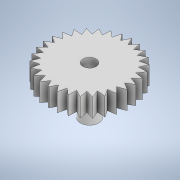
# Autodesk Inventor part: motor driven gear straight teeth for potentiometer
Saved by Autodesk Inventor 2022 (Build 260153000, 153)
## iProperties
Created: 2021-11-09
Part Number: motor driven gear straight teeth for potentiometer
Material: Generic
Document SubType Name: Modeling
Designer: a-dubs
Density: 1 g/cm^3
Appearance: Default
Author: a-dubs
Autodesk Inventor part; units mm, degrees
ref_plane "YZ Plane" through (0, 0, 0) normal (1, 0, 0) x (0, 1, 0)
ref_plane "XZ Plane" through (0, 0, 0) normal (0, 1, 0) x (-1, 0, 0)
ref_plane "XY Plane" through (0, 0, 0) normal (0, 0, 1) x (1, 0, 0)
sketch "Sketch1" plane through (0, 0, 0) normal (0, 1, 0) x (-1, 0, 0)
  line L0 (-2, 0) -> (2, 0)
  line L1 (-2, 0) -> (-2, 1)
  line L2 (-2, 1) -> (0, 0)
  line L3 (0, 0) -> (2, 1)
  line L4 (0, 0) -> (0, 19)
  line L5 (0, 19) -> (2, 19)
  line L6 (-2, 19) -> (0, 19)
  line L7 (0, 19) -> (0, 23)
  line L8 (0, 23) -> (-2, 19)
  line L9 (2, 19) -> (0, 23)
  line L10 (2, 0) -> (2, 19)
  line L11 (-2, 19) -> (-2, 0)
  point P0 (0, 41)
  dimension "d6" = 1
  dimension "d10" = 19
  dimension "d11" = 4
  constraints: 24 end point, 2 equal length, 1 vertical
  measures "d6" distance of L0.start L1.end
  measures "d10" distance of L2.end L4.end
  measures "d11" distance of L4.end L7.end
extrude "Extrusion1" add sketch "Sketch1" along normal blind 26 contours L3 L10 L0 | L4 L5 L10 L3 | L2 L11 L6 L4 | L7 L9 L5 | L6 L8 L7
pattern_circular "Circular Pattern1" count 30 over 360 about axis through (0, 0, 0) along (0, 1, 0) of "Extrusion1"
fillet "Fillet1" radius 0.5 1 edges at (0, 13, 23)
sketch "Sketch2" plane through (0, 26, 0) normal (0, 1, 0) x (1, 0, 0)
  circle A0 centre (0, 0) radius 1.5
  circle A1 centre (0, 0) radius 2.8
  line L0 (0, 0) -> (0, 1.9)
  line L1 (0, 1.9) -> (0, -1.9)
  line L2 (0, -1.9) -> (-2.0567, -1.9)
  line L3 (0, -1.9) -> (2.0567, -1.9)
  line L4 (0, 1.9) -> (2.0567, 1.9)
  line L5 (0, 1.9) -> (-2.0567, 1.9)
  circle A2 centre (0, 0) radius 3.6
  line L6 (0, 0) -> (0, 0.7)
  line L7 (0, 0) -> (0, -0.7)
  circle A3 centre (0, 0) radius 2.9
  line L8 (0, 0.7) -> (-2.8142, 0.7)
  line L9 (0, -0.7) -> (-2.8142, -0.7)
  line L10 (0, -0.7) -> (2.8142, -0.7)
  line L11 (0, 0.7) -> (2.8142, 0.7)
  circle A4 centre (0, 0) radius 5
  circle A5 centre (0, 0) radius 15
  circle A6 centre (0, 0) radius 30.1844
  line L12 (-2.0567, 1.9) -> (-2.1909, 1.9)
  line L13 (-2.1909, -1.9) -> (-2.0567, -1.9)
  line L14 (2.0567, -1.9) -> (2.1909, -1.9)
  line L15 (2.0567, 1.9) -> (2.1909, 1.9)
  line L16 (-1.0864, -1.9) -> (-1.0864, -2)
  line L17 (-1.0864, 1.9) -> (-1.0864, 2)
  line L18 (-1.0864, 2) -> (-2.1, 2)
  line L19 (-1.0864, 2) -> (2.1, 2)
  line L20 (-2.1, -2) -> (-1.0864, -2)
  line L21 (-1.0864, -2) -> (2.1, -2)
  circle A7 centre (0, 0) radius 3
  point P0 (1.9596, -2)
  point P1 (-1.9596, -2)
  point P2 (1.9596, 2)
  point P3 (-1.9596, 2)
  dimension "d30" = 5.8
  dimension "d13" = 3
  dimension "d19" = 5.6
  dimension "d20" = 1.9
  dimension "d21" = 3.8
  dimension "d27" = 7.2
  dimension "d28" = 0.7
  dimension "d29" = 0.7
  dimension "d37" = 10
  dimension "d38" = 30
  dimension "d43" = 0.1
  dimension "d44" = 0.1
  dimension "d47" = 6
  constraints: 44 end point, 11 point on line, 8 coincident, 7 centre point, 5 parallel, 4 point on circle, 3 horizontal, 3 vertical, 1 perpendicular, 14 other
  measures "d13" diameter of A0
  measures "d19" diameter of A1
  measures "d20" distance of L0.start L0.end
  measures "d21" distance of L0.end L1.end
  measures "d27" diameter of A2
  measures "d28" distance of L6.start L6.end
  measures "d29" distance of L6.start L7.end
  measures "d37" diameter of A4
  measures "d38" diameter of A5
  measures "d43" distance of L16.start L16.end
  measures "d44" distance of L17.start L17.end
  measures "d47" diameter of A7
extrude "Extrusion2" cut sketch "Sketch2" against normal blind 7.5 contours A0 L10 L1 L0 L11 | A0 L11 A1 L10 | L11 L0 A0 | A0 L0 L4 A1 L11 | L10 A1 L3 L1 A0 | A0 L1 L10 | L0 L8 A0 | A0 L8 A1 L5 L0 | L0 L1 L9 A0 L8 | L11 A3 L10 A1 | A1 L15 A3 L11 | L1 L2 A1 L9 A0 | A0 L9 L1 | L10 A3 L14 A1 | A0 L9 A1 L8 | L5 L17 L19 A1 L4 | A1 L19 A3 L15 | L3 A1 L21 L16 L2 | L14 A3 L21 A1 | L8 A3 L12 A1 | A1 L9 A3 L8 | L5 A1 L18 L17 | L19 L18 A1 | A1 L18 A3 L19 | A1 L13 A3 L9 | L16 L20 A1 L2 | L21 A3 L20 A1 | A1 L20 L21 | L12 A3 L18 A1 | A1 L20 A3 L13 | A2 | A7
pattern_circular "Circular Pattern2" [suppressed]
extrude "Extrusion4" cut sketch "Sketch2" against normal blind 8.5 from surface at -7.5 contours A0 L10 L1 L0 L11 | A0 L11 A1 L10 | L11 L0 A0 | A0 L0 L4 A1 L11 | L10 A1 L3 L1 A0 | A0 L1 L10 | L0 L8 A0 | A0 L8 A1 L5 L0 | L0 L1 L9 A0 L8 | L11 A3 L10 A1 | A1 L15 A3 L11 | L1 L2 A1 L9 A0 | A0 L9 L1 | L10 A3 L14 A1 | A0 L9 A1 L8 | L5 L17 L19 A1 L4 | A1 L19 A3 L15 | L3 A1 L21 L16 L2 | L14 A3 L21 A1 | L8 A3 L12 A1 | A1 L9 A3 L8 | L5 A1 L18 L17 | L19 L18 A1 | A1 L18 A3 L19 | A1 L13 A3 L9 | L16 L20 A1 L2 | L21 A3 L20 A1 | A1 L20 L21 | L12 A3 L18 A1 | A1 L20 A3 L13 | A7
extrude "Extrusion6" cut sketch "Sketch2" along normal blind 10 from surface at -26 contours A0 L10 L1 L0 L11 | A0 L11 A1 L10 | L11 L0 A0 | A0 L0 L4 A1 L11 | L10 A1 L3 L1 A0 | A0 L1 L10 | L0 L8 A0 | A0 L8 A1 L5 L0 | L0 L1 L9 A0 L8 | L11 A3 L10 A1 | A1 L15 A3 L11 | L1 L2 A1 L9 A0 | A0 L9 L1 | L10 A3 L14 A1 | A0 L9 A1 L8 | L5 L17 L19 A1 L4 | L3 A1 L21 L16 L2 | L8 A3 L12 A1 | A1 L9 A3 L8 | L5 A1 L18 L17 | A1 L13 A3 L9 | L16 L20 A1 L2
extrude "Extrusion9" cut sketch "Sketch2" along normal blind 16 from surface at -26 contours A5 | A6
body "Solid1"
